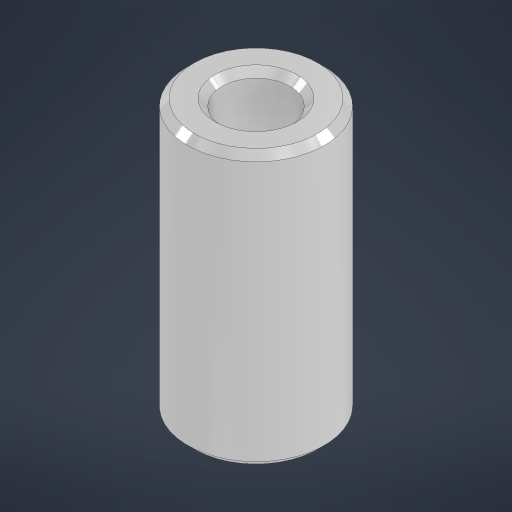
# Autodesk Inventor part: Practice_001_1inchspacer
Saved by Autodesk Inventor 2024.4 (Build 284460000, 460)
## iProperties
Created: 2026-06-08
Part Number: Practice_001_1inchspacer
Material: Aluminum 6061
Document SubType Name: Modeling
Designer: hs4ho
Density: 2.7 g/cm^3
Appearance: Aluminum - Polished
Author: hs4ho
Autodesk Inventor part; units mm, degrees
ref_plane "YZ Plane" through (0, 0, 0) normal (1, 0, 0) x (0, 1, 0)
ref_plane "XZ Plane" through (0, 0, 0) normal (0, 1, 0) x (-1, 0, 0)
ref_plane "XY Plane" through (0, 0, 0) normal (0, 0, 1) x (1, 0, 0)
sketch "Sketch1" plane through (0, 0, 0) normal (0, 1, 0) x (-1, 0, 0)
  circle A0 centre (0, 0) radius 6.35
  dimension "d0" = 12.7
  constraints: 1 centre point, 1 coincident
  measures "d0" diameter of A0
extrude "Extrusion1" add sketch "Sketch1" along normal blind 25.4
sketch "Sketch2" plane through (0, 25.4, 0) normal (0, 1, 0) x (1, 0, 0)
  point P0 (0, 0)
  point P1 (0, 0)
  constraints: 1 coincident
hole "Hole1" at (0, 25.4, 0) direction (0, -1, 0) diameter 6.35 end through all
chamfer "Chamfer1" distance 0.635 angle 45 2 edges at (6.35, 25.4, 0) (6.35, 0, 0)
chamfer "Chamfer2" distance 0.635 angle 45 2 edges at (0, 25.4, -3.175) (0, 0, -3.175)
body "Solid1"
